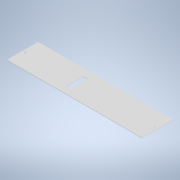
# Autodesk Inventor part: metal_cap_forPrint
Saved by Autodesk Inventor 2022 (Build 260153000, 153)
## iProperties
Created: 2024-12-12
Part Number: metal_cap_forPrint
Material: Типовые
Document SubType Name: Modeling
Designer: Andrey
Density: 1 g/cm^3
Appearance: По умолчанию
Author: Andrey
Autodesk Inventor part; units mm, degrees
ref_plane "YZ Plane" through (0, 0, 0) normal (1, 0, 0) x (0, 1, 0)
ref_plane "XZ Plane" through (0, 0, 0) normal (0, 1, 0) x (-1, 0, 0)
ref_plane "XY Plane" through (0, 0, 0) normal (0, 0, 1) x (1, 0, 0)
sketch "Эскиз1" plane through (0, 0, 0) normal (0, 1, 0) x (-1, 0, 0)
  circle A0 centre (169.2619, 20) radius 1.1
  line L0 (100.131, 30.85) -> (105.631, 30.85)
  line L1 (105.631, 30.85) -> (105.631, 9.15)
  line L2 (105.631, 9.15) -> (100.131, 9.15)
  line L3 (100.131, 9.15) -> (100.131, 30.85)
  arc A1 (0, 40) -> (-0.5, 39.5) centre (0, 39.5) ccw
  line L4 (-0.5, 0.5) -> (-0.5, 39.5)
  arc A2 (-0.5, 0.5) -> (0, 0) centre (0, 0.5) ccw
  line L5 (172.2619, 0) -> (0, 0)
  arc A3 (172.2619, 0) -> (172.7619, 0.5) centre (172.2619, 0.5) ccw
  line L6 (172.7619, 39.5) -> (172.7619, 0.5)
  arc A4 (172.7619, 39.5) -> (172.2619, 40) centre (172.2619, 39.5) ccw
  line L7 (0, 40) -> (172.2619, 40)
  circle A5 centre (3, 20) radius 1.1
  constraints: 16 end point, 8 point on circle, 6 centre point
extrude "Выдавливание1" add sketch "Эскиз1" along normal blind 0.5
